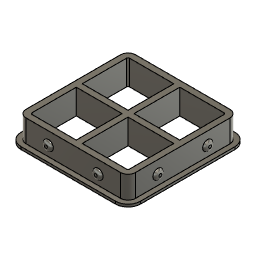
MontanaMaskFilterFrameWithFlange (Autodesk Fusion 360 design; units mm, degrees)
Autodesk Fusion 360 part; units mm, degrees
sketch "Sketch1" plane through (0, 0, 0) normal (0, 1, 0) x (1, 0, 0)
  arc A0 (20.7456, 20.8766) -> (17.7456, 23.8766) centre (17.7456, 20.8766) ccw
  line L0 (-20.2544, 23.8766) -> (17.7456, 23.8766)
  arc A1 (-20.2544, 23.8766) -> (-23.2544, 20.8766) centre (-20.2544, 20.8766) ccw
  line L1 (-23.2544, -17.1234) -> (-23.2544, 20.8766)
  arc A2 (-23.2544, -17.1234) -> (-20.2544, -20.1234) centre (-20.2544, -17.1234) ccw
  line L2 (17.7456, -20.1234) -> (-20.2544, -20.1234)
  arc A3 (17.7456, -20.1234) -> (20.7456, -17.1234) centre (17.7456, -17.1234) ccw
  line L3 (20.7456, 20.8766) -> (20.7456, -17.1234)
  arc A4 (18.3456, 20.8766) -> (17.7456, 21.4766) centre (17.7456, 20.8766) ccw
  line L4 (-20.2544, 21.4766) -> (17.7456, 21.4766)
  arc A5 (-20.2544, 21.4766) -> (-20.8544, 20.8766) centre (-20.2544, 20.8766) ccw
  line L5 (-20.8544, -17.1234) -> (-20.8544, 20.8766)
  arc A6 (-20.8544, -17.1234) -> (-20.2544, -17.7234) centre (-20.2544, -17.1234) ccw
  line L6 (17.7456, -17.7234) -> (-20.2544, -17.7234)
  arc A7 (17.7456, -17.7234) -> (18.3456, -17.1234) centre (17.7456, -17.1234) ccw
  line L7 (18.3456, 20.8766) -> (18.3456, -17.1234)
  line L8 (-2.4544, 21.4766) -> (-0.0544, 21.4766)
  line L9 (-0.0544, 21.4766) -> (-0.0544, -17.7234)
  line L10 (-0.0544, -17.7234) -> (-2.4544, -17.7234)
  line L11 (-2.4544, -17.7234) -> (-2.4544, 21.4766)
  line L12 (-20.8544, 3.0766) -> (18.3456, 3.0766)
  line L13 (18.3456, 3.0766) -> (18.3456, 0.6766)
  line L14 (18.3456, 0.6766) -> (-20.8544, 0.6766)
  line L15 (-20.8544, 0.6766) -> (-20.8544, 3.0766)
  dimension "d5" = 2.4
  dimension "d6" = 2.4
  dimension "d7" = 2.4
  dimension "d8" = 18.4
  dimension "d10" = 18.4
  constraint tangent L2 A3
  constraint tangent A0 L3
  constraint tangent A0 L0
  constraint tangent L0 A1
  constraint tangent L1 A2
  constraint tangent A1 L1
  constraint tangent A2 L2
  constraint tangent A3 L3
  constraint horizontal L8
  constraint vertical L9
  constraint horizontal L10
  constraint vertical L11
  constraint coincident L6 L9.end
  constraint coincident L4 L8.start
  constraint horizontal L12
  constraint vertical L13
  constraint horizontal L14
  constraint vertical L15
  constraint coincident L7 L13.end
  constraint coincident L5 L12.start
  measures "d6" distance of L12 L14
  measures "d7" distance of L9 L11
  measures "d8" distance of L6 L14
  measures "d10" distance of L7 L9
extrude "Extrude1" add sketch "Sketch1" along normal blind 10 contours A0 L0 A1 L1 A2 L2 A3 L3 | L7 L9 L12 L13 L14 | L4 L8 L9 L11 L12 | L9 L11 L12 L14 | L6 L9 L10 L11 L14 | L5 L11 L12 L14 L15
sketch "Sketch2" plane through (0, 0, 20.1234) normal (0, 0, 1) x (1, 0, 0)
  line L0 (-20.2544, 0) -> (17.7456, 0)
  line L1 (17.7456, 0) -> (17.7456, 10)
  line L2 (17.7456, 10) -> (-20.2544, 10)
  line L3 (-20.2544, 10) -> (-20.2544, 0)
  circle A0 centre (-11.2544, 5) radius 2
  circle A1 centre (8.7456, 5) radius 2
  line L4 (-23.2544, 0) -> (-23.2544, 10)
  line L5 (20.7456, 0) -> (20.7456, 10)
  dimension "d13" = 4
  dimension "d14" = 4
  dimension "d15" = 12
  dimension "d16" = 12
  dimension "d17" = 5
  dimension "d18" = 5
  measures "d13" diameter of A0
  measures "d14" diameter of A1
  measures "d15" distance of A0.centre L4
  measures "d16" distance of A1.centre L5
  measures "d17" distance of L0 A0.centre
  measures "d18" distance of L0 A1.centre
extrude "Extrude2" add sketch "Sketch2" along normal blind 1 contours A0 | A1
fillet "Fillet1" radius 1.5 2 edges at (-13.119, 4.2768, 21.1234) (6.881, 4.2768, 21.1234)
sketch "Sketch3" plane through (0, 0, -23.8766) normal (0, 0, -1) x (-1, 0, 0)
  line L0 (-17.7456, 0) -> (20.2544, 0)
  line L1 (20.2544, 0) -> (20.2544, 10)
  line L2 (20.2544, 10) -> (-17.7456, 10)
  line L3 (-17.7456, 10) -> (-17.7456, 0)
  circle A0 centre (-8.7456, 5) radius 2
  circle A1 centre (11.2544, 5) radius 2
  line L4 (23.2544, 0) -> (23.2544, 10)
  line L5 (-20.7456, 0) -> (-20.7456, 10)
  dimension "d22" = 4
  dimension "d23" = 4
  dimension "d24" = 12
  dimension "d25" = 12
  dimension "d26" = 5
  dimension "d27" = 5
  measures "d22" diameter of A0
  measures "d23" diameter of A1
  measures "d24" distance of A1.centre L4
  measures "d25" distance of A0.centre L5
  measures "d26" distance of L0 A0.centre
  measures "d27" distance of L0 A1.centre
extrude "Extrude3" add sketch "Sketch3" along normal blind 1 contours A0 | A1
fillet "Fillet2" radius 1.5 2 edges at (10.6103, 4.2768, -24.8766) (-9.3897, 4.2768, -24.8766)
sketch "Sketch4" plane through (-23.2544, 0, 0) normal (-1, 0, 0) x (0, 0, 1)
  line L0 (-20.8766, 0) -> (17.1234, 0)
  line L1 (17.1234, 0) -> (17.1234, 10)
  line L2 (17.1234, 10) -> (-20.8766, 10)
  line L3 (-20.8766, 10) -> (-20.8766, 0)
  circle A0 centre (-11.8766, 5) radius 2
  circle A1 centre (8.1234, 5) radius 2
  line L4 (-23.8766, 0) -> (-23.8766, 10)
  line L5 (20.1234, 0) -> (20.1234, 10)
  dimension "d31" = 4
  dimension "d32" = 4
  dimension "d33" = 12
  dimension "d34" = 12
  dimension "d35" = 5
  dimension "d36" = 5
  measures "d31" diameter of A0
  measures "d32" diameter of A1
  measures "d33" distance of A0.centre L4
  measures "d34" distance of A1.centre L5
  measures "d35" distance of L0 A1.centre
  measures "d36" distance of L0 A0.centre
extrude "Extrude4" add sketch "Sketch4" along normal blind 1 contours A0 | A1
fillet "Fillet3" radius 1.5 2 edges at (-24.2544, 4.2768, -13.7413) (-24.2544, 4.2768, 6.2587)
sketch "Sketch5" plane through (20.7456, 0, 0) normal (1, 0, 0) x (0, 0, -1)
  line L0 (-17.1234, 0) -> (20.8766, 0)
  line L1 (20.8766, 0) -> (20.8766, 10)
  line L2 (20.8766, 10) -> (-17.1234, 10)
  line L3 (-17.1234, 10) -> (-17.1234, 0)
  circle A0 centre (-8.1234, 5) radius 2
  circle A1 centre (11.8766, 5) radius 2
  line L4 (23.8766, 0) -> (23.8766, 10)
  line L5 (-20.1234, 0) -> (-20.1234, 10)
  dimension "d40" = 4
  dimension "d41" = 4
  dimension "d42" = 12
  dimension "d43" = 12
  dimension "d44" = 5
  dimension "d45" = 5
  measures "d40" diameter of A0
  measures "d41" diameter of A1
  measures "d42" distance of A1.centre L4
  measures "d43" distance of A0.centre L5
  measures "d44" distance of L0 A0.centre
  measures "d45" distance of L0 A1.centre
extrude "Extrude5" add sketch "Sketch5" along normal blind 1 contours A0 | A1
fillet "Fillet4" radius 1.5 2 edges at (21.7456, 4.2768, 9.9881) (21.7456, 4.2768, -10.0119)
sketch "Sketch6" plane through (0, 0, 0) normal (0, -1, 0) x (1, 0, 0)
  arc A0 (-20.8544, -20.8766) -> (-20.2544, -21.4766) centre (-20.2544, -20.8766) ccw
  line L0 (-20.8544, -20.8766) -> (-20.8544, -3.0766)
  line L1 (-20.8544, -3.0766) -> (-2.4544, -3.0766)
  line L2 (-2.4544, -3.0766) -> (-2.4544, -21.4766)
  line L3 (-2.4544, -21.4766) -> (-20.2544, -21.4766)
  arc A1 (-20.2544, 17.7234) -> (-20.8544, 17.1234) centre (-20.2544, 17.1234) ccw
  line L4 (-20.2544, 17.7234) -> (-2.4544, 17.7234)
  line L5 (-2.4544, 17.7234) -> (-2.4544, -0.6766)
  line L6 (-2.4544, -0.6766) -> (-20.8544, -0.6766)
  line L7 (-20.8544, -0.6766) -> (-20.8544, 17.1234)
  arc A2 (18.3456, 17.1234) -> (17.7456, 17.7234) centre (17.7456, 17.1234) ccw
  line L8 (18.3456, 17.1234) -> (18.3456, -0.6766)
  line L9 (18.3456, -0.6766) -> (-0.0544, -0.6766)
  line L10 (-0.0544, -0.6766) -> (-0.0544, 17.7234)
  line L11 (-0.0544, 17.7234) -> (17.7456, 17.7234)
  arc A3 (17.7456, -21.4766) -> (18.3456, -20.8766) centre (17.7456, -20.8766) ccw
  line L12 (17.7456, -21.4766) -> (-0.0544, -21.4766)
  line L13 (-0.0544, -21.4766) -> (-0.0544, -3.0766)
  line L14 (-0.0544, -3.0766) -> (18.3456, -3.0766)
  line L15 (18.3456, -3.0766) -> (18.3456, -20.8766)
  arc A4 (-23.2544, -20.8766) -> (-20.2544, -23.8766) centre (-20.2544, -20.8766) ccw
  line L16 (-20.2544, -23.8766) -> (17.7456, -23.8766)
  arc A5 (17.7456, -23.8766) -> (20.7456, -20.8766) centre (17.7456, -20.8766) ccw
  line L17 (20.7456, -20.8766) -> (20.7456, 17.1234)
  arc A6 (20.7456, 17.1234) -> (17.7456, 20.1234) centre (17.7456, 17.1234) ccw
  line L18 (17.7456, 20.1234) -> (-20.2544, 20.1234)
  arc A7 (-20.2544, 20.1234) -> (-23.2544, 17.1234) centre (-20.2544, 17.1234) ccw
  line L19 (-23.2544, 17.1234) -> (-23.2544, -20.8766)
  line L20 (-25.2544, 17.1234) -> (-25.2544, -20.8766)
  arc A8 (-25.2544, -20.8766) -> (-20.2544, -25.8766) centre (-20.2544, -20.8766) ccw
  line L21 (-20.2544, -25.8766) -> (17.7456, -25.8766)
  arc A9 (17.7456, -25.8766) -> (22.7456, -20.8766) centre (17.7456, -20.8766) ccw
  line L22 (22.7456, -20.8766) -> (22.7456, 17.1234)
  arc A10 (22.7456, 17.1234) -> (17.7456, 22.1234) centre (17.7456, 17.1234) ccw
  line L23 (17.7456, 22.1234) -> (-20.2544, 22.1234)
  arc A11 (-20.2544, 22.1234) -> (-25.2544, 17.1234) centre (-20.2544, 17.1234) ccw
  line L24 (-23.2544, 17.1234) -> (-23.2544, -20.8766)
  arc A12 (-23.2544, -20.8766) -> (-20.2544, -23.8766) centre (-20.2544, -20.8766) ccw
  line L25 (-20.2544, -23.8766) -> (17.7456, -23.8766)
  arc A13 (17.7456, -23.8766) -> (20.7456, -20.8766) centre (17.7456, -20.8766) ccw
  line L26 (20.7456, -20.8766) -> (20.7456, 17.1234)
  arc A14 (20.7456, 17.1234) -> (17.7456, 20.1234) centre (17.7456, 17.1234) ccw
  line L27 (17.7456, 20.1234) -> (-20.2544, 20.1234)
  arc A15 (-20.2544, 20.1234) -> (-23.2544, 17.1234) centre (-20.2544, 17.1234) ccw
  dimension "d49" = 2
  dimension "d50" = 0
  measures "d50" distance of L19
extrude "Extrude6" add sketch "Sketch6" against normal blind 1 contours L20 A8 L21 A9 L22 A10 L23 A11
